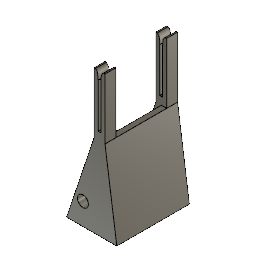
VerticalPerfusionStand (Autodesk Fusion 360 design; units mm, degrees)
Autodesk Fusion 360 part; units mm, degrees
sketch "Sketch1" plane through (0, 0, 0) normal (0, 1, 0) x (1, 0, 0)
  line L0 (-5, 0) -> (5, 0)
  line L1 (5, 0) -> (5, -55)
  line L2 (5, -55) -> (-5, -55)
  line L3 (-5, -55) -> (-5, 0)
  line L4 (1.25, -7) -> (-1.25, -7)
  line L5 (-1.25, -7) -> (-1.25, -47)
  line L6 (-1.25, -47) -> (1.25, -47)
  line L7 (1.25, -47) -> (1.25, -7)
  line L8 (1.25, -7) -> (-1.25, -47) construction
  line L9 (-1.25, -7) -> (1.25, -47) construction
  spline S0 degree 5 poles (1.25, -47) (1.257, -47.1229) (1.2709, -47.3671) (1.2914, -47.7288) (1.3183, -48.2018) (1.3512, -48.7775) (1.3843, -49.3372) (1.419, -49.8802) (1.4579, -50.4059) (1.5048, -50.9136) (1.5653, -51.4025) (1.6457, -51.8719) (1.7521, -52.3205) (1.8885, -52.7467) (2.0565, -53.148) (2.2527, -53.521) (2.4693, -53.8614) (2.6961, -54.1645) (2.9221, -54.4262) (3.1377, -54.6429) (3.3369, -54.8128) (3.4808, -54.9111) (3.5798, -54.9637) (3.6419, -54.9895) (3.6719, -55) knots 0 0 0 0 0 0 0.05 0.1 0.15 0.2 0.25 0.3 0.35 0.4 0.45 0.5 0.55 0.6 0.65 0.7 0.75 0.8 0.85 0.9 0.95 1 1 1 1 1 1
  line L10 (0, -50) -> (0, -52.5)
  spline S1 degree 5 poles (-1.25, -47) (-1.257, -47.1229) (-1.2709, -47.3671) (-1.2914, -47.7288) (-1.3183, -48.2018) (-1.3512, -48.7775) (-1.3843, -49.3372) (-1.419, -49.8802) (-1.4579, -50.4059) (-1.5048, -50.9136) (-1.5653, -51.4025) (-1.6457, -51.8719) (-1.7521, -52.3205) (-1.8885, -52.7467) (-2.0565, -53.148) (-2.2527, -53.521) (-2.4693, -53.8614) (-2.6961, -54.1645) (-2.9221, -54.4262) (-3.1377, -54.6429) (-3.3369, -54.8128) (-3.4808, -54.9111) (-3.5798, -54.9637) (-3.6419, -54.9895) (-3.6719, -55) knots 0 0 0 0 0 0 0.05 0.1 0.15 0.2 0.25 0.3 0.35 0.4 0.45 0.5 0.55 0.6 0.65 0.7 0.75 0.8 0.85 0.9 0.95 1 1 1 1 1 1
  line L11 (1.1935, -46.0048) -> (1.3065, -47.9952)
  line L12 (3.0882, -54.795) -> (4.2556, -55.205)
  line L13 (-1.1935, -46.0048) -> (-1.3065, -47.9952)
  line L14 (-3.0882, -54.795) -> (-4.2556, -55.205)
  line L15 (15.7143, 75) -> (-30, 75)
  line L16 (5, 0) -> (15.7143, 75)
  line L17 (-5, 0) -> (-30, 75)
  point P0 (0, -27)
  point P1 (1.4697, -50.5148)
  point P2 (2, -53)
  point P3 (3, -54.5)
  point P4 (-1.4697, -50.5148)
  point P5 (-2, -53)
  point P6 (-3, -54.5)
  dimension "d1" = 55
  dimension "d2" = 40
  dimension "d3" = 2.5
  constraint horizontal L0
  constraint vertical L1
  constraint horizontal L2
  constraint vertical L3
  constraint perpendicular L4 L5
  constraint parallel L4 L6
  constraint parallel L5 L7
  constraint horizontal L4
  constraint coincident L8 P0
  constraint coincident L9 P0
  constraint coincident L2 S0.end
  constraint perpendicular L6 L10
  constraint midpoint L6.end L11
  constraint midpoint S0.end L12
  constraint symmetric L6.end L10 L5.end
  constraint symmetric P1 L10 P4
  constraint symmetric P2 L10 P5
  constraint symmetric P3 L10 P6
  constraint symmetric S0.end L10 S1.end
  constraint symmetric L10 L11.start L13.start
  constraint symmetric L10 L11.end L13.end
  constraint symmetric L10 L12.start L14.start
  constraint symmetric L10 L12.end L14.end
  constraint horizontal L15
  measures "d1" distance of L0.start L2.end
  measures "d2" distance of L4.end L5.end
  measures "d3" distance of L5.end L6.end
extrude "Extrude1" add sketch "Sketch1" along normal blind 10 contours L0 L15 L16 L17 | L0 L1 L2 L3 L4 L5 L7 S0 S1 L11 L13 makes body 1
move_body "Move1" bodies 1 to x (1, 0, 0) y (0, 1, 0) z (0, 0, 1) at (0, 23, 0)
mirror "Mirror1" about plane through (0, 0, 0) normal (0, 1, 0) of bodies 1 makes body 2
sketch "Sketch2" plane through (0, -23, 0) normal (0, 1, 0) x (-1, 0, 0)
  spline S0 degree 5 poles (-1.25, 47) (-1.257, 47.1229) (-1.2709, 47.3671) (-1.2914, 47.7288) (-1.3183, 48.2018) (-1.3512, 48.7775) (-1.3843, 49.3372) (-1.419, 49.8802) (-1.4579, 50.4059) (-1.5048, 50.9136) (-1.5653, 51.4025) (-1.6457, 51.8719) (-1.7521, 52.3205) (-1.8885, 52.7467) (-2.0565, 53.148) (-2.2527, 53.521) (-2.4693, 53.8614) (-2.6961, 54.1645) (-2.9221, 54.4262) (-3.1377, 54.6429) (-3.3369, 54.8128) (-3.4808, 54.9111) (-3.5798, 54.9637) (-3.6419, 54.9895) (-3.6719, 55) knots 0 0 0 0 0 0 0.05 0.1 0.15 0.2 0.25 0.3 0.35 0.4 0.45 0.5 0.55 0.6 0.65 0.7 0.75 0.8 0.85 0.9 0.95 1 1 1 1 1 1
  line L0 (-3.6719, 55) -> (-5, 55)
  line L1 (-5, 55) -> (-5, 0)
  line L2 (-5, 0) -> (-15.7143, -75)
  line L3 (-15.7143, -75) -> (30, -75)
  line L4 (30, -75) -> (5, 0)
  line L5 (5, 0) -> (5, 55)
  line L6 (5, 55) -> (3.6719, 55)
  spline S1 degree 5 poles (1.25, 47) (1.257, 47.1229) (1.2709, 47.3671) (1.2914, 47.7288) (1.3183, 48.2018) (1.3512, 48.7775) (1.3843, 49.3372) (1.419, 49.8802) (1.4579, 50.4059) (1.5048, 50.9136) (1.5653, 51.4025) (1.6457, 51.8719) (1.7521, 52.3205) (1.8885, 52.7467) (2.0565, 53.148) (2.2527, 53.521) (2.4693, 53.8614) (2.6961, 54.1645) (2.9221, 54.4262) (3.1377, 54.6429) (3.3369, 54.8128) (3.4808, 54.9111) (3.5798, 54.9637) (3.6419, 54.9895) (3.6719, 55) knots 0 0 0 0 0 0 0.05 0.1 0.15 0.2 0.25 0.3 0.35 0.4 0.45 0.5 0.55 0.6 0.65 0.7 0.75 0.8 0.85 0.9 0.95 1 1 1 1 1 1
  line L7 (1.25, 47) -> (1.25, 7)
  line L8 (1.25, 7) -> (-1.25, 7)
  line L9 (-1.25, 7) -> (-1.25, 47)
  line L10 (-0.0825, 0) -> (-10.7967, -75)
  line L11 (-0.0825, 0) -> (-5, 0)
  line L12 (26.7345, -65.2034) -> (-14.3148, -65.2034)
  constraint coincident L3 L10.end
  constraint parallel L2 L10
  constraint coincident L1.end L2.start
  constraint horizontal L11
  constraint coincident L4 L12.start
  constraint coincident L2 L12.end
  constraint horizontal L12
extrude "Extrude2" add sketch "Sketch2" along normal up to near side of body 1 contours L2 L10 L11 L12 | L2 L3 L10 L12 | L3 L4 L10 L12 bodies 1 2
sketch "Sketch3" plane through (0, 33, 0) normal (0, 1, 0) x (-1, 0, 0)
  spline S0 degree 5 poles (-1.25, 47) (-1.257, 47.1229) (-1.2709, 47.3671) (-1.2914, 47.7288) (-1.3183, 48.2018) (-1.3512, 48.7775) (-1.3843, 49.3372) (-1.419, 49.8802) (-1.4579, 50.4059) (-1.5048, 50.9136) (-1.5653, 51.4025) (-1.6457, 51.8719) (-1.7521, 52.3205) (-1.8885, 52.7467) (-2.0565, 53.148) (-2.2527, 53.521) (-2.4693, 53.8614) (-2.6961, 54.1645) (-2.9221, 54.4262) (-3.1377, 54.6429) (-3.3369, 54.8128) (-3.4808, 54.9111) (-3.5798, 54.9637) (-3.6419, 54.9895) (-3.6719, 55) knots 0 0 0 0 0 0 0.05 0.1 0.15 0.2 0.25 0.3 0.35 0.4 0.45 0.5 0.55 0.6 0.65 0.7 0.75 0.8 0.85 0.9 0.95 1 1 1 1 1 1
  line L0 (-3.6719, 55) -> (-5, 55)
  line L1 (-5, 55) -> (-5, 0)
  line L2 (30, -75) -> (5, 0)
  line L3 (5, 0) -> (5, 55)
  line L4 (5, 55) -> (3.6719, 55)
  spline S1 degree 5 poles (3.6719, 55) (3.6419, 54.9895) (3.5798, 54.9637) (3.4808, 54.9111) (3.3369, 54.8128) (3.1377, 54.6429) (2.9221, 54.4262) (2.6961, 54.1645) (2.4693, 53.8614) (2.2527, 53.521) (2.0565, 53.148) (1.8885, 52.7467) (1.7521, 52.3205) (1.6457, 51.8719) (1.5653, 51.4025) (1.5048, 50.9136) (1.4579, 50.4059) (1.419, 49.8802) (1.3843, 49.3372) (1.3512, 48.7775) (1.3183, 48.2018) (1.2914, 47.7288) (1.2709, 47.3671) (1.257, 47.1229) (1.25, 47) knots -1 -1 -1 -1 -1 -1 -0.95 -0.9 -0.85 -0.8 -0.75 -0.7 -0.65 -0.6 -0.55 -0.5 -0.45 -0.4 -0.35 -0.3 -0.25 -0.2 -0.15 -0.1 -0.05 0 0 0 0 0 0
  line L5 (1.25, 47) -> (1.25, 7)
  line L6 (1.25, 7) -> (-1.25, 7)
  line L7 (-1.25, 7) -> (-1.25, 47)
  line L8 (-5, 0) -> (-15.7143, -75)
  line L9 (-15.7143, -75) -> (30, -75)
  line L10 (26.7345, -65.2034) -> (-9.3972, -65.2034)
  circle A0 centre (15, -55) radius 5
  dimension "d12" = 10
  measures "d12" diameter of A0
extrude "Extrude3" cut sketch "Sketch3" against normal blind 88 contours A0 bodies 1
